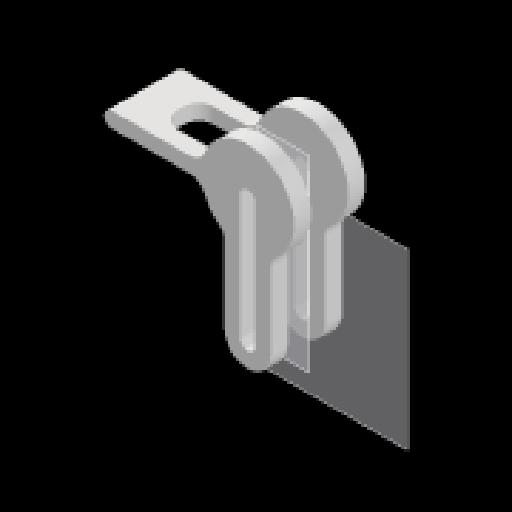
# Autodesk Inventor part: odomHousing
Saved by Autodesk Inventor 2024.1 (Build 281209000, 209)
## iProperties
Created: 2025-05-24
Part Number: odomHousing
Material: Generic
Document SubType Name: Modeling
Designer: Teddy
Density: 1 g/cm^3
Appearance: Default
Author: Teddy
Autodesk Inventor part; units mm, degrees
ref_plane "YZ Plane" through (0, 0, 0) normal (1, 0, 0) x (0, 1, 0)
ref_plane "XZ Plane" through (0, 0, 0) normal (0, 1, 0) x (-1, 0, 0)
ref_plane "XY Plane" through (0, 0, 0) normal (0, 0, 1) x (1, 0, 0)
ref_plane "Work Plane1" through (0, 0, 0) normal (0, 0, 1) x (1, 0, 0)
sketch "Sketch1" plane through (0, 0, 0) normal (0, 0, 1) x (1, 0, 0)
  circle A0 centre (0, 0) radius 3.175 projected
  line L0 (0, 0) -> (0, 50.8) construction
  line L1 (3.175, 0) -> (3.175, 50.8)
  line L2 (-3.175, 50.8) -> (-3.175, 0)
  arc A1 (-3.175, 0) -> (3.175, 0) centre (0, 0) ccw
  arc A2 (3.175, 50.8) -> (-3.175, 50.8) centre (0, 50.8) ccw
  line L3 (9.525, 50.8) -> (9.525, 0)
  arc A3 (-9.525, 0) -> (9.525, 0) centre (0, 0) ccw
  line L4 (-9.525, 0) -> (-9.525, 50.8)
  arc A4 (9.525, 50.8) -> (-9.525, 50.8) centre (0, 50.8) ccw
  circle A5 centre (0, 50.8) radius 19.05
  line L5 (0, 50.8) -> (-55.2684, 50.8) construction
  line L6 (0, 47.625) -> (-55.2684, 47.625)
  line L7 (-55.2684, 53.975) -> (0, 53.975)
  arc A6 (0, 47.625) -> (0, 53.975) centre (0, 50.8) ccw
  arc A7 (-55.2684, 53.975) -> (-55.2684, 47.625) centre (-55.2684, 50.8) ccw
  point P0 (0, 0)
  point P1 (0, 25.4)
  point P2 (-3.175, 0)
  point P3 (9.525, 34.3022)
  point P4 (-9.525, 34.3022)
  point P5 (-27.6342, 50.8)
  point P6 (-18.7836, 47.625)
  point P7 (-18.7836, 53.975)
  dimension "d0" = 50.8
  dimension "d1" = 6.35
  dimension "d6" = 38.1
  constraints: 20 end point, 12 point on circle, 8 tangent, 7 centre point, 3 parallel, 2 midpoint, 1 coincident, 1 horizontal, 1 vertical, 3 other
  measures "d0" distance of L0.start L0.end
  measures "d1" distance between parallel lines of L1 L3
  measures "d6" diameter of A5
extrude "Extrusion1" add sketch "Sketch1" along normal blind 34.29 contours L1 A5 L3 A3 L4 L2 A0 | L1 A2 L7 A4 L3 A5 | A5 L4 L6 L2 | L3 A4 L7 A5 | L6 L4 A4 L7 A2 L2 | A5 L6 L4 | L6 A5 L7 A4 L4 | L6 A7 L7 A5
ref_plane "Work Plane2" through (0, 0, 17.145) normal (0, 0, 1) x (1, 0, 0)
sketch "Sketch2" plane through (0, 0, 17.145) normal (0, 0, 1) x (1, 0, 0)
  line L0 (9.525, 0) -> (9.525, 34.3022) projected
  arc A0 (-9.525, 0) -> (9.525, 0) centre (0, 0) ccw projected
  line L1 (-9.525, 34.3022) -> (-9.525, 0) projected
  arc A1 (3.175, 50.8) -> (-3.175, 50.8) centre (0, 50.8) ccw projected
  line L2 (-3.175, 0) -> (-3.175, 50.8) projected
  arc A2 (-3.175, 0) -> (3.175, 0) centre (0, 0) ccw projected
  line L3 (3.175, 50.8) -> (3.175, 0) projected
  arc A3 (-18.7836, 47.625) -> (-9.525, 34.3022) centre (0, 50.8) ccw projected
  line L4 (0, 0) -> (0, 50.8) construction
  line L5 (-9.525, 0) -> (-9.525, 50.8)
  line L6 (9.525, 50.8) -> (9.525, 0)
  arc A4 (-9.525, 0) -> (9.525, 0) centre (0, 0) ccw
  arc A5 (9.525, 50.8) -> (-9.525, 50.8) centre (0, 50.8) ccw
  line L7 (-55.2684, 47.625) -> (-18.7836, 47.625) projected
  arc A6 (-55.2684, 53.975) -> (-55.2684, 47.625) centre (-55.2684, 50.8) ccw projected
  line L8 (-18.7836, 53.975) -> (-55.2684, 53.975) projected
  arc A7 (9.525, 34.3022) -> (-18.7836, 53.975) centre (0, 50.8) ccw projected
  circle A8 centre (0, 50.8) radius 19.05
  line L9 (-55.2684, 47.625) -> (-18.7836, 47.625) projected
  line L10 (-42.2273, 47.625) -> (-42.2273, 53.975)
  point P0 (0, 0)
  point P1 (0, 25.4)
  point P2 (9.525, 34.3022)
  constraints: 10 end point, 4 point on circle, 4 tangent, 3 centre point, 2 concentric, 2 point on line, 1 coincident, 1 midpoint, 1 parallel, 1 perpendicular, 1 vertical
extrude "Extrusion2" cut sketch "Sketch2" along normal mid plane 19.05 contours A0 L1 A8 L2 A2 L3 L0 | A8 L3 A1 L2 L5 A5 L6 | L6 A5 L5 A3 A8 A7 | A8 L7 L10 L8
fillet "Fillet1" radius 6.35 10 edges at (-42.2273, 50.8, 7.62) (-42.2273, 50.8, 26.67) (-18.7836, 53.975, 30.48) (-18.7836, 47.625, 30.48) (9.525, 34.3022, 3.81) (9.525, 34.3022, 30.48) (-18.7836, 53.975, 3.81) (-9.525, 34.3022, 30.48) (-9.525, 34.3022, 3.81) (-18.7836, 47.625, 3.81)
body "Solid1"
